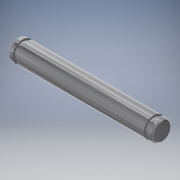
# Autodesk Inventor part: Component 25 (Rocker Arm Axle)
Saved by Autodesk Inventor 2018 (Build 220112000, 112)
## iProperties
Created: 2023-03-25
Part Number: Component 25 (Rocker Arm Axle)
Material: Generic
Document SubType Name: Modeling
Designer: Habib Mohamed
Density: 1 g/cm^3
Appearance: Aluminum - Polished
Author: Habib Mohamed
Autodesk Inventor part; units mm, degrees
ref_plane "YZ Plane" through (0, 0, 0) normal (1, 0, 0) x (0, 1, 0)
ref_plane "XZ Plane" through (0, 0, 0) normal (0, 1, 0) x (-1, 0, 0)
ref_plane "XY Plane" through (0, 0, 0) normal (0, 0, 1) x (1, 0, 0)
sketch "Sketch1" plane through (0, 0, 0) normal (0, 0, 1) x (1, 0, 0)
  line L0 (-14.15, 0) -> (14.15, 0)
  line L1 (14.15, 0) -> (14.15, 1.5)
  line L2 (13.65, 2) -> (13.15, 2)
  line L3 (13.15, 2) -> (13.15, 1.6)
  line L4 (13.15, 1.6) -> (12.5, 1.6)
  line L5 (12.5, 1.6) -> (12.5, 2)
  line L6 (12.5, 2) -> (-12.5, 2)
  line L7 (-12.5, 2) -> (-12.5, 1.6)
  line L8 (-12.5, 1.6) -> (-13.15, 1.6)
  line L9 (-13.15, 1.6) -> (-13.15, 2)
  line L10 (-13.15, 2) -> (-13.65, 2)
  line L11 (-14.15, 1.5) -> (-14.15, 0)
  arc A0 (-13.65, 2) -> (-14.15, 1.5) centre (-13.65, 1.5) ccw
  arc A1 (14.15, 1.5) -> (13.65, 2) centre (13.65, 1.5) ccw
  point P0 (0, 0)
  point P1 (14.15, 2)
  point P2 (-14.15, 2)
  point P3 (0, 0)
  dimension "d0" = 25
  dimension "d1" = 0.65
  dimension "d2" = 1
  dimension "d3" = 2
  dimension "d4" = 1.6
  dimension "d5" = 1.6
  dimension "d6" = 0.5
  dimension "d7" = 1
  dimension "d8" = 0.5
  constraints: 24 end point, 8 perpendicular, 8 point on line, 4 point on circle, 4 tangent, 2 centre point, 1 coincident, 1 collinear, 1 horizontal, 1 midpoint, 1 vertical
  measures "d0" distance of L5.end L6.end
  measures "d1" distance of L7.end L8.end
  measures "d2" distance of L9.end point (-14.15, 2)
  measures "d3" distance of L0.end point (14.15, 2)
  measures "d4" distance between parallel lines of L4 L0
  measures "d5" distance between parallel lines of L0 L8
  measures "d6" radius of A0
  measures "d7" distance of point (14.15, 2) L2.end
  measures "d8" radius of A1
revolve "Revolution1" add sketch "Sketch1" angle 360 about axis through (-14.15, 0, 0) along (1, 0, 0)
equation "\"d5\" = d4"
body "Solid1"
